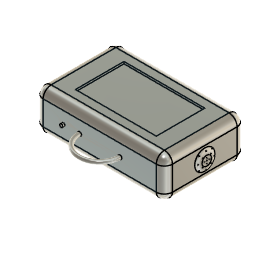
boot_prelim (Autodesk Fusion 360 design; units mm, degrees)
part number: 2025-10-20-15-09-19-256
Autodesk Fusion 360 part; units mm, degrees
sketch "Sketch1" plane through (0, 0, 0) normal (0, 0, 1) x (1, 0, 0)
  line L0 (-60, 30) -> (60, 30)
  line L1 (60, 30) -> (60, -30)
  line L2 (60, -30) -> (-60, -30)
  line L3 (-60, -30) -> (-60, 30)
  line L4 (-70, 50) -> (70, 50)
  line L5 (80, 40) -> (80, -40)
  line L6 (70, -50) -> (-70, -50)
  line L7 (-80, -40) -> (-80, 40)
  arc A0 (-70, 50) -> (-80, 40) centre (-70, 40) ccw
  arc A1 (80, 40) -> (70, 50) centre (70, 40) ccw
  arc A2 (70, -50) -> (80, -40) centre (70, -40) ccw
  arc A3 (-80, -40) -> (-70, -50) centre (-70, -40) ccw
  dimension "d1" = 10
  constraint horizontal L0
  constraint vertical L1
  constraint horizontal L2
  constraint vertical L3
  constraint horizontal L4
  constraint vertical L5
  constraint horizontal L6
  constraint vertical L7
  constraint tangent L4 A0
  constraint tangent L7 A0
  constraint tangent L4 A1
  constraint tangent L5 A1
  constraint equal A0 A1
  constraint tangent L5 A2
  constraint tangent L6 A2
  constraint equal A0 A2
  constraint tangent L6 A3
  constraint tangent L7 A3
  constraint equal A0 A3
  measures "d1" radius of A0
extrude "Extrude1" add sketch "Sketch1" along normal blind 50 contours L0 L1 L2 L3 | L4 L5 L6 L7 A0 A1 A2 A3
fillet "Fillet1" radius 10 8 edges at (77.0711, 47.0711, 0) (80, 0, 0) (77.0711, -47.0711, 0) (0, -50, 0) (-77.0711, -47.0711, 0) (-80, 0, 0) (-77.0711, 47.0711, 0) (0, 50, 0)
fillet "Fillet2" radius 10 8 edges at (-80, 0, 50) (-77.0711, -47.0711, 50) (0, -50, 50) (77.0711, -47.0711, 50) (80, 0, 50) (77.0711, 47.0711, 50) (0, 50, 50) (-77.0711, 47.0711, 50)
sketch "Sketch2" plane through (0, 0, 50) normal (0, 0, 1) x (-1, 0, 0)
  line L0 (70, -40) -> (70, 40)
  line L1 (70, 40) -> (-70, 40)
  line L2 (-70, 40) -> (-70, -40)
  line L3 (-70, -40) -> (70, -40)
  line L4 (-50, 30) -> (50, 30)
  line L5 (50, 30) -> (50, -30)
  line L6 (50, -30) -> (-50, -30)
  line L7 (-50, -30) -> (-50, 30)
  constraint horizontal L4
  constraint vertical L5
  constraint horizontal L6
  constraint vertical L7
extrude "Extrude2" cut sketch "Sketch2" against normal blind 2.5 contours L4 L5 L6 L7
sketch "Sketch3" plane through (80, 0, 0) normal (1, 0, 0) x (0, 1, 0)
  line L0 (40, 40) -> (-40, 40)
  line L1 (-40, 40) -> (-40, 10)
  line L2 (-40, 10) -> (40, 10)
  line L3 (40, 10) -> (40, 40)
  circle A0 centre (0, 25) radius 12.5
extrude "Extrude3" add sketch "Sketch3" along normal blind 2.5 contours A0
fillet "Fillet3" radius 10 1 edges at (82.5, -11.6541, 20.4798)
sketch "Sketch4" plane through (-80, 0, 0) normal (-1, 0, 0) x (0, -1, 0)
  line L0 (40, 40) -> (-40, 40)
  line L1 (-40, 40) -> (-40, 10)
  line L2 (-40, 10) -> (40, 10)
  line L3 (40, 10) -> (40, 40)
  line L4 (5, 15) -> (-5, 15)
  line L5 (-5, 15) -> (-5, 35)
  line L6 (-5, 35) -> (5, 35)
  line L7 (5, 35) -> (5, 15)
  constraint horizontal L4
  constraint vertical L5
  constraint horizontal L6
  constraint vertical L7
extrude "Extrude4" add sketch "Sketch4" along normal blind 5 contours L4 L5 L6 L7
sketch "Sketch5" plane through (0, 5, 0) normal (0, 1, 0) x (-1, 0, 0)
  line L0 (80, 35) -> (80, 15)
  line L1 (80, 15) -> (85, 15)
  line L2 (85, 15) -> (85, 35)
  line L3 (85, 35) -> (80, 35)
  arc A0 (80, 35) -> (85, 15) centre (122.5, 35) ccw
  constraint tangent L0 A0
  constraint coincident L0.start L3.end
  constraint coincident L1.end L2.start
extrude "Extrude5" cut sketch "Sketch5" against normal blind 10 contours L2 L3 A0
sketch "Sketch6" plane through (0, -50, 0) normal (0, -1, 0) x (1, 0, 0)
  line L0 (70, 40) -> (-70, 40)
  line L1 (-70, 40) -> (-70, 10)
  line L2 (-70, 10) -> (70, 10)
  line L3 (70, 10) -> (70, 40)
sketch "Sketch7" plane through (0, -50, 0) normal (0, -1, 0) x (1, 0, 0)
sketch "Sketch8" plane through (0, 0, 50) normal (0, 0, 1) x (-1, 0, 0)
  line L0 (50, 30) -> (50, -30)
  line L1 (50, -30) -> (-50, -30)
  line L2 (-50, -30) -> (-50, 30)
  line L3 (-50, 30) -> (50, 30)
  line L4 (70, -40) -> (70, 40)
  line L5 (70, 40) -> (-70, 40)
  line L6 (-70, 40) -> (-70, -40)
  line L7 (-70, -40) -> (70, -40)
sketch "Sketch9" plane through (0, -50, 0) normal (0, -1, 0) x (1, 0, 0)
sketch "Sketch10" plane through (0, 0, 0) normal (0, 1, 0) x (1, 0, 0)
sketch "Sketch11" plane through (0, 0, 50) normal (0, 0, 1) x (-1, 0, 0)
sketch "Sketch12" plane through (0, 0, 50) normal (0, 0, 1) x (-1, 0, 0)
sketch "Sketch13" plane through (0, -50, 0) normal (0, -1, 0) x (1, 0, 0)
  circle A0 centre (25, 25) radius 2.5
  circle A1 centre (-25, 25) radius 2.5
  line L0 (0, 10) -> (0, 40)
  dimension "d22" = 5
  dimension "d23" = 5
  constraint vertical L0
  measures "d22" diameter of A0
  measures "d23" diameter of A1
revolve "Revolve1" add sketch "Sketch13" angle 360 about axis through (0, -50, 10) along (0, 0, 1) contours A1
sketch "Sketch14" plane through (0, -50, 0) normal (0, -1, 0) x (1, 0, 0)
  circle A0 centre (-45, 25) radius 2
extrude "Extrude6" add sketch "Sketch14" along normal blind 2.5
sketch "Sketch15" plane through (82.5, 0, 0) normal (1, 0, 0) x (0, 1, 0)
  circle A0 centre (0, 25) radius 5.8856
  circle A1 centre (0, 25) radius 0.5
  circle A2 centre (0, 28) radius 0.5
  circle A3 centre (3, 25) radius 0.5
  circle A4 centre (0, 22) radius 0.5
  circle A5 centre (-3, 25) radius 0.5
  circle A6 centre (0, 35) radius 0.5
  circle A7 centre (10, 25) radius 0.5
  circle A8 centre (0, 15) radius 0.5
  circle A9 centre (-10, 25) radius 0.5
  circle A10 centre (-5, 30) radius 0.5
  circle A11 centre (-8, 33) radius 0.5
  circle A12 centre (5, 30) radius 0.5
  circle A13 centre (8, 33) radius 0.5
  circle A14 centre (5, 20) radius 0.5
  circle A15 centre (8, 17) radius 0.5
  circle A16 centre (-5, 20) radius 0.5
  circle A17 centre (-8, 17) radius 0.5
  dimension "d27" = 1
  dimension "d28" = 1
  dimension "d29" = 1
  dimension "d30" = 1
  dimension "d31" = 1
  dimension "d32" = 1
  dimension "d33" = 1
  dimension "d34" = 1
  dimension "d35" = 1
  dimension "d36" = 1
  dimension "d37" = 1
  dimension "d38" = 1
  dimension "d39" = 1
  dimension "d40" = 1
  dimension "d41" = 1
  dimension "d42" = 1
  dimension "d43" = 1
  constraint concentric A0 A1
  measures "d27" diameter of A1
  measures "d28" diameter of A2
  measures "d29" diameter of A3
  measures "d30" diameter of A4
  measures "d31" diameter of A5
  measures "d32" diameter of A6
  measures "d33" diameter of A7
  measures "d34" diameter of A8
  measures "d35" diameter of A9
  measures "d36" diameter of A10
  measures "d37" diameter of A11
  measures "d38" diameter of A12
  measures "d39" diameter of A13
  measures "d40" diameter of A14
  measures "d41" diameter of A15
  measures "d42" diameter of A16
  measures "d43" diameter of A17
extrude "Extrude7" cut sketch "Sketch15" against normal blind 6 contours A1 | A2 | A3 | A4 | A5 | A6 | A7 | A8 | A9 | A10 | A11 | A12 | A13 | A14 | A15 | A16 | A17
